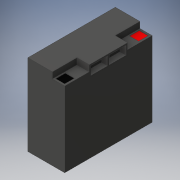
# Autodesk Inventor part: Battery-1111-2017
Saved by Autodesk Inventor 2016 SP2 (Build 200236200, 236)
## iProperties
Created: 2017-03-04
Part Number: Battery-1111-2017
Material: Generic
Document SubType Name: Modeling
Designer: smiku
Mass: 2242.42 g
Surface Area: 1215.39 cm^2
Volume: 2242.42 cm^3
Density: 1 g/cm^3
Appearance: Smooth - Dark Gray
Author: smiku
Autodesk Inventor part; units mm, degrees
ref_plane "YZ Plane" through (0, 0, 0) normal (1, 0, 0) x (0, 1, 0)
ref_plane "XZ Plane" through (0, 0, 0) normal (0, 1, 0) x (-1, 0, 0)
ref_plane "XY Plane" through (0, 0, 0) normal (0, 0, 1) x (1, 0, 0)
sketch "Sketch1" plane through (0, 0, 0) normal (0, 1, 0) x (-1, 0, 0)
  line L0 (0, 0) -> (76.2, 0)
  line L1 (76.2, 0) -> (76.2, -180.975)
  line L2 (76.2, -180.975) -> (0, -180.975)
  line L3 (0, -180.975) -> (0, 0)
  dimension "d0" = 76.2
  dimension "d1" = 180.975
  constraints: 8 end point, 2 parallel, 1 horizontal, 1 perpendicular
  measures "d0" distance of L1.end L2.end
  measures "d1" distance of L0.end L1.end
extrude "Extrusion1" add sketch "Sketch1" along normal blind 168.275
sketch "Sketch2" plane through (0, 168.275, 0) normal (0, 1, 0) x (1, 0, 0)
  line L0 (-76.2, 0) -> (0, 0) construction
  line L1 (0, 0) -> (0, 180.975) construction
  line L2 (0, 180.975) -> (-76.2, 180.975) construction
  line L3 (-76.2, 180.975) -> (-76.2, 0) construction
  line L4 (0, 0) -> (0, 180.975) projected
  line L5 (0, 0) -> (-25.4, 0)
  line L6 (-25.4, 0) -> (-25.4, 50.8)
  line L7 (-25.4, 50.8) -> (0, 50.8)
  line L8 (0, 50.8) -> (0, 0)
  line L9 (0, 180.975) -> (-25.4, 180.975)
  line L10 (-25.4, 180.975) -> (-25.4, 130.175)
  line L11 (-25.4, 130.175) -> (0, 130.175)
  line L12 (0, 130.175) -> (0, 180.975)
  dimension "d4" = 25.4
  dimension "d5" = 50.8
  dimension "d6" = 25.4
  dimension "d7" = 50.8
  constraints: 16 end point, 4 parallel, 2 horizontal, 2 perpendicular
  measures "d4" distance of L6.end L7.end
  measures "d5" distance of L5.end L6.end
  measures "d6" distance of L11.end L10.end
  measures "d7" distance of L10.end L9.end
extrude "Extrusion2" cut sketch "Sketch2" against normal blind 12.7
sketch "Sketch3" plane through (0, 0, 0) normal (1, 0, 0) x (0, 0, -1)
  line L0 (50.8, 168.275) -> (130.175, 168.275) construction
  line L1 (130.175, 155.575) -> (130.175, 168.275) construction
  line L2 (50.8, 168.275) -> (50.8, 155.575) construction
  line L3 (127, 155.575) -> (127, 165.1) construction
  line L4 (127, 165.1) -> (53.975, 165.1) construction
  line L5 (53.975, 165.1) -> (53.975, 155.575) construction
  line L6 (53.975, 165.1) -> (88.9, 165.1)
  line L7 (88.9, 165.1) -> (88.9, 147.32)
  line L8 (88.9, 147.32) -> (53.975, 147.32)
  line L9 (53.975, 147.32) -> (53.975, 165.1)
  line L10 (127, 165.1) -> (92.075, 165.1)
  line L11 (92.075, 165.1) -> (92.075, 147.32)
  line L12 (92.075, 147.32) -> (127, 147.32)
  line L13 (127, 147.32) -> (127, 165.1)
  point P0 (0, 0)
  dimension "d10" = 3.175
  dimension "d11" = 34.925
  dimension "d12" = 17.78
  dimension "d13" = 34.925
  dimension "d14" = 17.78
  dimension "d15" = 3.175
  constraints: 22 end point, 4 parallel, 2 horizontal, 2 perpendicular, 2 other
  measures "d10" distance between parallel lines of L0 L4
  measures "d11" distance of L7.end L8.end
  measures "d12" distance of L6.end L7.end
  measures "d13" distance of L12.end L11.end
  measures "d14" distance of L11.end L10.end
  measures "d15" distance between parallel lines of L11 L7
extrude "Extrusion3" cut sketch "Sketch3" against normal blind 12.7
sketch "Sketch4" plane through (0, 155.575, 0) normal (0, 1, 0) x (1, 0, 0)
  line L0 (0, 0) -> (-25.4, 0) construction
  line L1 (0, 50.8) -> (0, 0) construction
  line L2 (0, 180.975) -> (0, 130.175) construction
  line L3 (-25.4, 180.975) -> (0, 180.975) construction
  line L4 (-3.81, 50.8) -> (-3.81, 3.81) construction
  line L5 (-3.81, 3.81) -> (-25.4, 3.81) construction
  line L6 (-3.81, 130.175) -> (-3.81, 177.165) construction
  line L7 (-3.81, 177.165) -> (-25.4, 177.165) construction
  line L8 (-3.81, 3.81) -> (-22.86, 3.81)
  line L9 (-22.86, 3.81) -> (-22.86, 24.13)
  line L10 (-22.86, 24.13) -> (-3.81, 24.13)
  line L11 (-3.81, 24.13) -> (-3.81, 3.81)
  line L12 (-3.81, 177.165) -> (-22.86, 177.165)
  line L13 (-22.86, 177.165) -> (-22.86, 156.845)
  line L14 (-22.86, 156.845) -> (-3.81, 156.845)
  line L15 (-3.81, 156.845) -> (-3.81, 177.165)
  dimension "d18" = 3.81
  dimension "d19" = 3.81
  dimension "d20" = 19.05
  dimension "d21" = 20.32
  dimension "d22" = 19.05
  dimension "d23" = 20.32
  constraints: 24 end point, 4 parallel, 2 horizontal, 2 perpendicular, 2 other
  measures "d18" distance between parallel lines of L1 L4
  measures "d19" distance between parallel lines of L2 L6
  measures "d20" distance of L9.end L10.end
  measures "d21" distance of L8.end L9.end
  measures "d22" distance of L14.end L13.end
  measures "d23" distance of L13.end L12.end
extrude "Extrusion4" cut sketch "Sketch4" against normal blind 0.635
sketch "Sketch5" plane through (-76.2, 0, -180.975) normal (-1, 0, 0) x (0, 0, 1)
  line L0 (0, 168.275) -> (180.975, 168.275) construction
  line L1 (2.549, 165.1) -> (183.524, 165.1) construction
  line L2 (0, 0) -> (0, 168.275) construction
  line L3 (180.975, 0) -> (180.975, 168.275) construction
  line L4 (22.86, 2.1972) -> (22.86, 168.275) construction
  line L5 (158.115, 168.275) -> (158.115, 0) construction
  line L6 (22.86, 165.1) -> (66.04, 165.1)
  line L7 (66.04, 165.1) -> (66.04, 147.32)
  line L8 (66.04, 147.32) -> (22.86, 147.32)
  line L9 (22.86, 147.32) -> (22.86, 165.1)
  line L10 (158.115, 165.1) -> (114.935, 165.1)
  line L11 (114.935, 165.1) -> (114.935, 147.32)
  line L12 (114.935, 147.32) -> (158.115, 147.32)
  line L13 (158.115, 147.32) -> (158.115, 165.1)
  line L14 (66.04, 165.1) -> (69.215, 165.1) construction
  line L15 (114.935, 165.1) -> (111.76, 165.1) construction
  line L16 (69.215, 165.1) -> (111.76, 165.1)
  line L17 (111.76, 165.1) -> (111.76, 147.32)
  line L18 (111.76, 147.32) -> (69.215, 147.32)
  line L19 (69.215, 147.32) -> (69.215, 165.1)
  dimension "d26" = 3.175
  dimension "d27" = 22.86
  dimension "d28" = 22.86
  dimension "d29" = 43.18
  dimension "d30" = 43.18
  dimension "d31" = 17.78
  dimension "d32" = 3.175
  dimension "d33" = 3.175
  dimension "d34" = 42.545
  dimension "d35" = 17.78
  constraints: 34 end point, 8 point on line, 7 parallel, 3 perpendicular, 2 collinear, 2 horizontal
  measures "d26" distance between parallel lines of L0 L1
  measures "d27" distance between parallel lines of L2 L4
  measures "d28" distance between parallel lines of L5 L3
  measures "d29" distance of L7.end L8.end
  measures "d30" distance of L12.end L11.end
  measures "d31" distance of L6.end L7.end
  measures "d32" distance of L6.end L14.end
  measures "d33" distance of L10.end L15.end
  measures "d34" distance of L17.end L18.end
  measures "d35" distance of L15.end L17.end
extrude "Extrusion5" cut sketch "Sketch5" against normal blind 12.7
body "Solid1"
